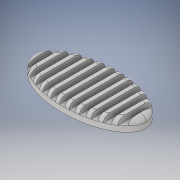
# Autodesk Inventor part: 示範二
Saved by Autodesk Inventor 2017 (Build 210142000, 142)
## iProperties
Part Number: 示範二
Material: 一般
Document SubType Name: Modeling
Designer: user
Density: 1 g/cm^3
Appearance: 預設
Author: user
Autodesk Inventor part; units mm, degrees
ref_plane "YZ Plane" through (0, 0, 0) normal (1, 0, 0) x (0, 1, 0)
ref_plane "XZ Plane" through (0, 0, 0) normal (0, 1, 0) x (-1, 0, 0)
ref_plane "XY Plane" through (0, 0, 0) normal (0, 0, 1) x (1, 0, 0)
sketch "草圖1" plane through (0, 0, 0) normal (0, 1, 0) x (-1, 0, 0)
  ellipse E0 centre (0, 0) end of major axis (-10, 0) minor radius 5
  dimension "d0" = 10
  dimension "d1" = 5
  constraints: 1 coincident, 2 other
extrude "擠出1" add sketch "草圖1" along normal blind 2
fillet "圓角1" radius 1 1 edges at (-10, 2, 0)
sketch "草圖2" plane through (0, 0, 0) normal (0, 0, 1) x (1, 0, 0)
  line L0 (-9, 2) -> (-9, 1)
  line L1 (-9, 1) -> (-8, 1)
  line L2 (-8, 1) -> (-8, 2)
  line L3 (-8, 2) -> (-9, 2)
  line L4 (-10, 0) -> (10, 0) projected
  line L5 (-10, 0) -> (-10, 3.2236)
  point P0 (0, 0)
  dimension "d5" = 2
  dimension "d6" = 1
  dimension "d7" = 1
  dimension "d8" = 2
  constraints: 10 end point, 3 perpendicular, 2 vertical
  measures "d5" diameter of L0 L5
  measures "d6" distance of L2.end L0.start
  measures "d7" distance between parallel lines of L1 L4
  measures "d8" distance from line of L3 L4.start
extrude "擠出2" cut sketch "草圖2" against normal up to next
sketch "草圖3" plane through (0, 0, 0) normal (0, 0, -1) x (-1, 0, 0)
  line L0 (9, 2) -> (9, 1) projected
  line L1 (8, 2) -> (9, 2) projected
  line L2 (8, 1) -> (8, 2) projected
  line L3 (9, 1) -> (8, 1) projected
  point P0 (0, 0)
extrude "擠出3" cut sketch "草圖3" against normal up to next
sketch "草圖4" plane through (0, 2, 0) normal (0, 1, 0) x (1, 0, 0)
  line L0 (-7.3, 11.742) -> (-7.3, -8.258)
  ellipse E0 centre (0, 0) end of major axis (-10, 0) minor radius 5 projected
  line L1 (-7.3, -8.258) -> (-6.3, -8.258)
  line L2 (-6.3, -8.258) -> (-6.3, 11.742)
  line L3 (-6.3, 11.742) -> (-7.3, 11.742)
  line L4 (-9, -2.1794) -> (-9, 2.1794) projected
  line L5 (-11.0785, -28.258) -> (12.7198, -28.258)
  line L6 (0, 0) -> (-13.0078, 0)
  line L7 (-5.6, 11.742) -> (-5.6, -8.258)
  line L8 (-4.6, -8.258) -> (-4.6, 11.742)
  line L9 (-4.6, 11.742) -> (-5.6, 11.742)
  line L10 (-5.6, -8.258) -> (-4.6, -8.258)
  line L11 (-3.9, 11.742) -> (-3.9, -8.258)
  line L12 (-2.9, -8.258) -> (-2.9, 11.742)
  line L13 (-2.9, 11.742) -> (-3.9, 11.742)
  line L14 (-3.9, -8.258) -> (-2.9, -8.258)
  line L15 (-2.2, 11.742) -> (-2.2, -8.258)
  line L16 (-1.2, -8.258) -> (-1.2, 11.742)
  line L17 (-1.2, 11.742) -> (-2.2, 11.742)
  line L18 (-2.2, -8.258) -> (-1.2, -8.258)
  line L19 (-0.5, 11.742) -> (-0.5, -8.258)
  line L20 (0.5, -8.258) -> (0.5, 11.742)
  line L21 (0.5, 11.742) -> (-0.5, 11.742)
  line L22 (-0.5, -8.258) -> (0.5, -8.258)
  line L23 (1.2, 11.742) -> (1.2, -8.258)
  line L24 (2.2, -8.258) -> (2.2, 11.742)
  line L25 (2.2, 11.742) -> (1.2, 11.742)
  line L26 (1.2, -8.258) -> (2.2, -8.258)
  line L27 (2.9, 11.742) -> (2.9, -8.258)
  line L28 (3.9, -8.258) -> (3.9, 11.742)
  line L29 (3.9, 11.742) -> (2.9, 11.742)
  line L30 (2.9, -8.258) -> (3.9, -8.258)
  line L31 (4.6, 11.742) -> (4.6, -8.258)
  line L32 (5.6, -8.258) -> (5.6, 11.742)
  line L33 (5.6, 11.742) -> (4.6, 11.742)
  line L34 (4.6, -8.258) -> (5.6, -8.258)
  line L35 (6.3, 11.742) -> (6.3, -8.258)
  line L36 (7.3, -8.258) -> (7.3, 11.742)
  line L37 (7.3, 11.742) -> (6.3, 11.742)
  line L38 (6.3, -8.258) -> (7.3, -8.258)
  line L39 (8, 11.742) -> (8, -8.258)
  line L40 (9, -8.258) -> (9, 11.742)
  line L41 (9, 11.742) -> (8, 11.742)
  line L42 (8, -8.258) -> (9, -8.258)
  dimension "d17" = 1.7
  dimension "d18" = 1
  dimension "d19" = 20
  dimension "d22" = 1.7
  constraints: 84 end point, 3 horizontal, 3 perpendicular, 1 vertical, 74 other
  measures "d17" distance between parallel lines of L0 L4
  measures "d18" distance of L2.end L0.start
  measures "d19" distance of L1.end L2.end
  measures "d22" distance of L0.start L7.start
extrude "擠出4" cut sketch "草圖4" against normal blind 1 contours L3 L2 E0 L0 | E0 L2 L6 L0 | L6 L2 E0 L0 | E0 L2 L1 L0 | L7 L9 L8 E0 | E0 L8 L6 L7 | L6 L8 E0 L7 | E0 L8 L10 L7 | L11 L13 L12 E0 | E0 L12 L6 L11 | L6 L12 E0 L11 | E0 L12 L14 L11 | L15 L17 L16 E0 | E0 L16 L6 L15 | L6 L16 E0 L15 | E0 L16 L18 L15 | L19 L21 L20 E0 | E0 L20 L19 | E0 L20 L22 L19 | L23 L25 L24 E0 | E0 L24 L23 | E0 L24 L26 L23 | L27 L29 L28 E0 | E0 L28 L27 | E0 L28 L30 L27 | L31 L33 L32 E0 | E0 L32 L31 | E0 L32 L34 L31 | L35 L37 L36 E0 | E0 L36 L35 | E0 L36 L38 L35 | L39 L41 L40 E0 | E0 L40 L39 | E0 L40 L42 L39
sketch "草圖5" plane through (0, 1, 0) normal (0, 1, 0) x (1, 0, 0)
  point P0 (0, 0)
